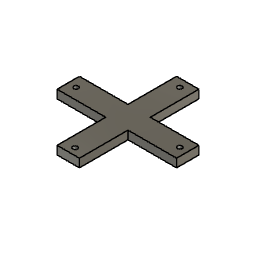
Base gripper v1 (Autodesk Fusion 360 design; units mm, degrees)
Autodesk Fusion 360 part; units mm, degrees
note: some values were not read from the file. Set by a fixed rule: which face or edge a step refers to.
sketch "Esboço1" plane through (0, 0, 0) normal (0, 0, 1) x (1, 0, 0)
  line L0 (12, 64.25) -> (-12, 64.25)
  line L1 (-12, 64.25) -> (-12, -64.25)
  line L2 (-12, -64.25) -> (12, -64.25)
  line L3 (12, -64.25) -> (12, 64.25)
  line L4 (12, 64.25) -> (-12, -64.25) construction
  line L5 (-12, 64.25) -> (12, -64.25) construction
  line L6 (64.25, 12) -> (-64.25, 12)
  line L7 (-64.25, 12) -> (-64.25, -12)
  line L8 (-64.25, -12) -> (64.25, -12)
  line L9 (64.25, -12) -> (64.25, 12)
  line L10 (64.25, 12) -> (-64.25, -12) construction
  line L11 (-64.25, 12) -> (64.25, -12) construction
  circle A0 centre (0, 0) radius 1.5
  line L12 (40, 1) -> (-40, 1)
  line L13 (-40, 1) -> (-40, -1)
  line L14 (-40, -1) -> (40, -1)
  line L15 (40, -1) -> (40, 1)
  line L16 (40, 1) -> (-40, -1) construction
  line L17 (-40, 1) -> (40, -1) construction
  line L18 (1, 40) -> (-1, 40)
  line L19 (-1, 40) -> (-1, -40)
  line L20 (-1, -40) -> (1, -40)
  line L21 (1, -40) -> (1, 40)
  line L22 (1, 40) -> (-1, -40) construction
  line L23 (-1, 40) -> (1, -40) construction
  line L24 (46.5, 6.5) -> (-46.5, 6.5)
  line L25 (-46.5, 6.5) -> (-46.5, -6.5)
  line L26 (-46.5, -6.5) -> (46.5, -6.5)
  line L27 (46.5, -6.5) -> (46.5, 6.5)
  line L28 (46.5, 6.5) -> (-46.5, -6.5) construction
  line L29 (-46.5, 6.5) -> (46.5, -6.5) construction
  line L30 (6.5, 46.5) -> (-6.5, 46.5)
  line L31 (-6.5, 46.5) -> (-6.5, -46.5)
  line L32 (-6.5, -46.5) -> (6.5, -46.5)
  line L33 (6.5, -46.5) -> (6.5, 46.5)
  line L34 (6.5, 46.5) -> (-6.5, -46.5) construction
  line L35 (-6.5, 46.5) -> (6.5, -46.5) construction
  line L36 (-64.25, 12) -> (64.25, 12)
  line L37 (64.25, 12) -> (64.25, 10)
  line L38 (64.25, 10) -> (-64.25, 10)
  line L39 (-64.25, 10) -> (-64.25, 12)
  line L40 (-64.25, -12) -> (64.25, -12)
  line L41 (64.25, -12) -> (64.25, -10)
  line L42 (64.25, -10) -> (-64.25, -10)
  line L43 (-64.25, -10) -> (-64.25, -12)
  line L44 (-64.25, 12) -> (-62.25, 12)
  line L45 (-62.25, 12) -> (-62.25, -12)
  line L46 (-62.25, -12) -> (-64.25, -12)
  line L47 (-64.25, -12) -> (-64.25, 12)
  line L48 (64.25, 12) -> (62.25, 12)
  line L49 (62.25, 12) -> (62.25, -12)
  line L50 (62.25, -12) -> (64.25, -12)
  line L51 (64.25, -12) -> (64.25, 12)
  line L52 (-12, 64.25) -> (-10, 64.25)
  line L53 (-10, 64.25) -> (-10, 10)
  line L54 (-10, 10) -> (-12, 10)
  line L55 (-12, 10) -> (-12, 64.25)
  line L56 (12, 64.25) -> (-12, 64.25)
  line L57 (-12, 64.25) -> (-12, 62.25)
  line L58 (-12, 62.25) -> (12, 62.25)
  line L59 (12, 62.25) -> (12, 64.25)
  line L60 (12, 64.25) -> (10, 64.25)
  line L61 (10, 64.25) -> (10, 12)
  line L62 (10, 12) -> (12, 12)
  line L63 (12, 12) -> (12, 64.25)
  line L64 (-12, -64.25) -> (-10, -64.25)
  line L65 (-10, -64.25) -> (-10, -10)
  line L66 (-10, -10) -> (-12, -10)
  line L67 (-12, -10) -> (-12, -64.25)
  line L68 (12, -64.25) -> (10, -64.25)
  line L69 (10, -64.25) -> (10, -10)
  line L70 (10, -10) -> (12, -10)
  line L71 (12, -10) -> (12, -64.25)
  line L72 (-12, -64.25) -> (12, -64.25)
  line L73 (12, -64.25) -> (12, -62.25)
  line L74 (12, -62.25) -> (-12, -62.25)
  line L75 (-12, -62.25) -> (-12, -64.25)
  line L76 (10, 12) -> (10, 10)
  dimension "d1" = 24
  dimension "d2" = 128.5
  dimension "d3" = 128.5
  dimension "d4" = 24
  dimension "d5" = 3
  dimension "d6" = 80
  dimension "d7" = 2
  dimension "d8" = 80
  dimension "d11" = 93
  dimension "d12" = 13
  dimension "d13" = 13
  dimension "d14" = 93
  dimension "d15" = 2
  dimension "d16" = 2
  dimension "d17" = 2
  dimension "d18" = 2
  dimension "d19" = 2
  dimension "d20" = 2
  dimension "d21" = 2
  dimension "d22" = 2
  dimension "d23" = 2
  constraint horizontal L0
  constraint perpendicular L0 L1
  constraint parallel L0 L2
  constraint parallel L1 L3
  constraint coincident L4 A0.centre
  constraint coincident L5 A0.centre
  constraint coincident A0.centre origin
  constraint horizontal L6
  constraint perpendicular L6 L7
  constraint parallel L6 L8
  constraint parallel L7 L9
  constraint coincident L10 A0.centre
  constraint coincident L11 A0.centre
  constraint horizontal L12
  constraint perpendicular L12 L13
  constraint parallel L12 L14
  constraint parallel L13 L15
  constraint coincident L16 A0.centre
  constraint coincident L17 A0.centre
  constraint horizontal L18
  constraint perpendicular L18 L19
  constraint parallel L18 L20
  constraint parallel L19 L21
  constraint coincident L22 A0.centre
  constraint coincident L23 A0.centre
  constraint horizontal L24
  constraint perpendicular L24 L25
  constraint parallel L24 L26
  constraint parallel L25 L27
  constraint coincident L28 A0.centre
  constraint coincident L29 A0.centre
  constraint horizontal L30
  constraint perpendicular L30 L31
  constraint parallel L30 L32
  constraint parallel L31 L33
  constraint coincident L34 A0.centre
  constraint coincident L35 A0.centre
  constraint horizontal L36
  constraint vertical L37
  constraint horizontal L38
  constraint vertical L39
  constraint horizontal L40
  constraint vertical L41
  constraint horizontal L42
  constraint vertical L43
  constraint horizontal L44
  constraint vertical L45
  constraint horizontal L46
  constraint vertical L47
  constraint horizontal L48
  constraint vertical L49
  constraint horizontal L50
  constraint vertical L51
  constraint horizontal L52
  constraint vertical L53
  constraint horizontal L54
  constraint vertical L55
  constraint coincident L38 L53.end
  constraint horizontal L56
  constraint vertical L57
  constraint horizontal L58
  constraint vertical L59
  constraint horizontal L60
  constraint vertical L61
  constraint horizontal L62
  constraint vertical L63
  constraint horizontal L64
  constraint vertical L65
  constraint horizontal L66
  constraint vertical L67
  constraint horizontal L68
  constraint vertical L69
  constraint horizontal L70
  constraint vertical L71
  constraint horizontal L72
  constraint vertical L73
  constraint horizontal L74
  constraint vertical L75
  constraint coincident L38 L76.end
  constraint perpendicular L38 L76
  measures "d1" distance of L0.start L0.end
  measures "d2" distance of L0.start L2.end
  measures "d3" distance of L7.end L8.end
  measures "d4" distance of L6.start L8.end
  measures "d5" diameter of A0
  measures "d6" distance of L13.end L14.end
  measures "d7" distance of L12.start L14.end
  measures "d8" distance of L18.end L19.end
  measures "d11" distance of L25.end L26.end
  measures "d12" distance of L24.end L25.end
  measures "d13" distance of L30.start L30.end
  measures "d14" distance of L30.start L32.end
  measures "d15" distance of L6.end L38.end
  measures "d16" distance of L7.end L42.end
  measures "d17" distance of L6.end L44.end
  measures "d18" distance of L6.start L48.end
  measures "d19" distance of L0.start L58.end
  measures "d20" distance of L0.start L60.end
  measures "d21" distance of L1.end L64.end
  measures "d22" distance of L2.end L68.end
  measures "d23" distance of L1.end L74.end
extrude "Extrusão1" add sketch "Esboço1" along normal blind 2 makes body 1
extrude "Extrusão2" add sketch "Esboço1" against normal blind 3 contours L6 L30 L31 L33 L36 L53 L58 L61 | L6 L33 L36 L38 L76 | L3 L24 L26 L27 L38 L42 L49 | L3 L24 L33 L38 | L6 L31 L36 L38 L53 | L1 L24 L31 L38 L54 | L1 L24 L25 L26 L38 L42 L45 | L3 L26 L33 L42 L70 | L8 L33 L40 L42 L69 | L8 L31 L32 L33 L40 L65 L69 L74 | L1 L26 L31 L42 L66 | L8 L31 L40 L42 L65 bodies 1
extrude "Extrusão3" add sketch "Esboço1" against normal blind 6 contours L0 L3 L56 L58 L59 L60 L61 L63 | L0 L53 L56 L58 L61 | L3 L6 L36 L58 L61 L62 L63 | L0 L1 L52 L53 L55 L56 L57 L58 | L3 L6 L36 L38 L49 | L3 L6 L36 L38 L62 L76 | L1 L6 L36 L53 L55 L58 | L6 L9 L36 L37 L38 L48 L49 L51 | L1 L6 L36 L38 L53 L54 L55 | L9 L38 L42 L49 L51 | L1 L6 L36 L38 L45 L55 | L3 L8 L40 L42 L49 L71 | L8 L9 L40 L41 L42 L49 L50 L51 | L6 L7 L36 L38 L39 L44 L45 L47 | L3 L8 L40 L42 L69 L70 L71 | L7 L38 L42 L45 L47 | L3 L8 L40 L69 L71 L74 | L7 L8 L40 L42 L43 L45 L46 L47 | L1 L8 L40 L42 L45 L67 | L2 L3 L68 L69 L71 L72 L73 L74 | L1 L8 L40 L42 L65 L66 L67 | L2 L65 L69 L72 L74 | L1 L8 L40 L65 L67 L74 | L1 L2 L64 L65 L67 L72 L74 L75 bodies 1
sketch "Esboço2" plane through (0, 0, 0) normal (0, 0, -1) x (1, 0, 0)
  line L0 (6.5, 46.5) -> (-6.5, 46.5)
  line L1 (-6.5, 46.5) -> (-6.5, 6.5)
  line L2 (-6.5, 6.5) -> (-46.5, 6.5)
  line L3 (-46.5, 6.5) -> (-46.5, -6.5)
  line L4 (-46.5, -6.5) -> (-6.5, -6.5)
  line L5 (-6.5, -6.5) -> (-6.5, -46.5)
  line L6 (-6.5, -46.5) -> (6.5, -46.5)
  line L7 (6.5, -46.5) -> (6.5, -6.5)
  line L8 (6.5, -6.5) -> (46.5, -6.5)
  line L9 (46.5, -6.5) -> (46.5, 6.5)
  line L10 (46.5, 6.5) -> (6.5, 6.5)
  line L11 (6.5, 6.5) -> (6.5, 46.5)
  line L12 (3, 45) -> (-3, 45)
  line L13 (-3, 45) -> (-3, -45)
  line L14 (-3, -45) -> (3, -45)
  line L15 (3, -45) -> (3, 45)
  line L16 (3, 45) -> (-3, -45) construction
  line L17 (-3, 45) -> (3, -45) construction
  line L18 (45, 3) -> (-45, 3)
  line L19 (-45, 3) -> (-45, -3)
  line L20 (-45, -3) -> (45, -3)
  line L21 (45, -3) -> (45, 3)
  line L22 (45, 3) -> (-45, -3) construction
  line L23 (-45, 3) -> (45, -3) construction
  line L24 (-3, 3) -> (-3, 10) construction
  line L25 (0, 0) -> (0, 75) construction
  line L26 (0, 0) -> (0, -75) construction
  line L27 (0, 0) -> (-80, 0) construction
  line L28 (0, 0) -> (91.9976, 0) construction
  line L29 (-3, 10) -> (0, 10) construction
  line L30 (5, -67.1453) -> (-5, -67.1453) construction
  line L31 (-5, -67.1453) -> (-5, 67.1453) construction
  line L32 (-5, 67.1453) -> (5, 67.1453) construction
  line L33 (5, 67.1453) -> (5, -67.1453)
  line L34 (5, -67.1453) -> (-5, 67.1453) construction
  line L35 (-5, -67.1453) -> (5, 67.1453) construction
  line L36 (80.4505, 5) -> (-80.4505, 5) construction
  line L37 (-80.4505, 5) -> (-80.4505, -5) construction
  line L38 (-80.4505, -5) -> (80.4505, -5) construction
  line L39 (80.4505, -5) -> (80.4505, 5) construction
  line L40 (80.4505, 5) -> (-80.4505, -5) construction
  line L41 (-80.4505, 5) -> (80.4505, -5) construction
  line L42 (-5, 3) -> (-5, 10) construction
  line L43 (-5, 10) -> (5, 10)
  line L44 (5, 10) -> (5, 15)
  line L45 (5, 15) -> (-5, 15)
  line L46 (-5, 15) -> (-5, 10)
  line L47 (-5, 15) -> (5, 10) construction
  line L48 (5, 13.5) -> (-5, 13.5)
  line L49 (-5, 13.5) -> (-5, 11.5)
  line L50 (-5, 11.5) -> (5, 11.5)
  line L51 (5, 11.5) -> (5, 13.5)
  line L52 (5, 13.5) -> (-5, 11.5) construction
  line L53 (-5, 13.5) -> (5, 11.5) construction
  line L54 (-5, 15) -> (-5, 18.2)
  line L55 (-5, 18.2) -> (5, 18.2)
  line L56 (5, 18.2) -> (5, 23.7)
  line L57 (5, 23.7) -> (-5, 23.7)
  line L58 (-5, 23.7) -> (-5, 18.2)
  line L59 (5, 22.25) -> (-5, 22.25)
  line L60 (-5, 22.25) -> (-5, 19.75)
  line L61 (-5, 19.75) -> (5, 19.75)
  line L62 (5, 19.75) -> (5, 22.25)
  line L63 (5, 22.25) -> (-5, 19.75) construction
  line L64 (-5, 22.25) -> (5, 19.75) construction
  line L65 (-5, 23.7) -> (-5, 27.5)
  line L66 (-5, 27.5) -> (5, 27.5)
  line L67 (5, 27.5) -> (5, 32.5)
  line L68 (5, 32.5) -> (-5, 32.5)
  line L69 (-5, 32.5) -> (-5, 27.5)
  line L70 (5, 31.25) -> (-5, 31.25)
  line L71 (-5, 31.25) -> (-5, 28.75)
  line L72 (-5, 28.75) -> (5, 28.75)
  line L73 (5, 28.75) -> (5, 31.25)
  line L74 (5, 31.25) -> (-5, 28.75) construction
  line L75 (-5, 31.25) -> (5, 28.75) construction
  line L76 (-5, 32.5) -> (-5, 36.5)
  line L77 (-5, 36.5) -> (5, 36.5)
  line L78 (5, 36.5) -> (5, 44)
  line L79 (5, 44) -> (-5, 44)
  line L80 (-5, 44) -> (-5, 36.5)
  line L81 (-5, 44) -> (5, 36.5) construction
  line L82 (5, 43.25) -> (-5, 43.25)
  line L83 (-5, 43.25) -> (-5, 37.25)
  line L84 (-5, 37.25) -> (5, 37.25)
  line L85 (5, 37.25) -> (5, 43.25)
  line L86 (5, 43.25) -> (-5, 37.25) construction
  line L87 (-5, 43.25) -> (5, 37.25) construction
  line L88 (45, 1.5) -> (-45, 1.5)
  line L89 (-45, 1.5) -> (-45, -1.5)
  line L90 (-45, -1.5) -> (45, -1.5)
  line L91 (45, -1.5) -> (45, 1.5)
  line L92 (45, 1.5) -> (-45, -1.5) construction
  line L93 (-45, 1.5) -> (45, -1.5) construction
  line L94 (1.5, 45) -> (-1.5, 45)
  line L95 (-1.5, 45) -> (-1.5, -45)
  line L96 (-1.5, -45) -> (1.5, -45)
  line L97 (1.5, -45) -> (1.5, 45)
  line L98 (1.5, 45) -> (-1.5, -45) construction
  line L99 (-1.5, 45) -> (1.5, -45) construction
  point P0 (0, 12.5)
  point P1 (0, 21)
  point P2 (0, 30)
  point P3 (0, 40.25)
  dimension "d28" = 6
  dimension "d29" = 90
  dimension "d30" = 90
  dimension "d31" = 7
  dimension "d33" = 6
  dimension "d34" = 10
  dimension "d35" = 10
  dimension "d36" = 5
  dimension "d37" = 2
  dimension "d38" = 3.2
  dimension "d39" = 5.5
  dimension "d40" = 2.5
  dimension "d41" = 3.8
  dimension "d42" = 5
  dimension "d43" = 2.5
  dimension "d44" = 4
  dimension "d45" = 7.5
  dimension "d46" = 6
  dimension "d47" = 3
  dimension "d48" = 3
  constraint horizontal L12
  constraint perpendicular L12 L13
  constraint parallel L12 L14
  constraint parallel L13 L15
  constraint coincident L16 L25.start
  constraint coincident L17 L25.start
  constraint coincident L25.start L26.start
  constraint horizontal L18
  constraint perpendicular L18 L19
  constraint parallel L18 L20
  constraint parallel L19 L21
  constraint coincident L22 L25.start
  constraint coincident L23 L25.start
  constraint coincident L13 L24.start
  constraint coincident L18 L24.start
  constraint perpendicular L18 L24
  constraint perpendicular L12 L25
  constraint parallel L15 L26
  constraint perpendicular L3 L27
  constraint perpendicular L9 L28
  constraint coincident L25 L29.end
  constraint perpendicular L25 L29
  constraint horizontal L30
  constraint perpendicular L30 L31
  constraint parallel L30 L32
  constraint parallel L31 L33
  constraint coincident L34 L25.start
  constraint coincident L35 L25.start
  constraint horizontal L36
  constraint perpendicular L36 L37
  constraint parallel L36 L38
  constraint parallel L37 L39
  constraint coincident L40 L25.start
  constraint coincident L41 L25.start
  constraint coincident L18 L42.start
  constraint coincident L31 L42.start
  constraint coincident L31 L42.end
  constraint horizontal L43
  constraint vertical L44
  constraint horizontal L45
  constraint vertical L46
  constraint horizontal L48
  constraint perpendicular L48 L49
  constraint parallel L48 L50
  constraint parallel L49 L51
  constraint coincident L52 P0
  constraint coincident L53 P0
  constraint midpoint L47 P0
  constraint perpendicular L45 L54
  constraint horizontal L55
  constraint vertical L56
  constraint horizontal L57
  constraint vertical L58
  constraint horizontal L59
  constraint perpendicular L59 L60
  constraint parallel L59 L61
  constraint parallel L60 L62
  constraint coincident L63 P1
  constraint coincident L64 P1
  constraint coincident L25 P1
  constraint perpendicular L57 L65
  constraint horizontal L66
  constraint vertical L67
  constraint horizontal L68
  constraint vertical L69
  constraint horizontal L70
  constraint perpendicular L70 L71
  constraint parallel L70 L72
  constraint parallel L71 L73
  constraint coincident L74 P2
  constraint coincident L75 P2
  constraint coincident L67 L70.start
  constraint coincident L33 L70.start
  constraint coincident L25 P2
  constraint perpendicular L68 L76
  constraint horizontal L77
  constraint vertical L78
  constraint horizontal L79
  constraint vertical L80
  constraint horizontal L82
  constraint perpendicular L82 L83
  constraint parallel L82 L84
  constraint parallel L83 L85
  constraint coincident L86 P3
  constraint coincident L87 P3
  constraint coincident L78 L82.start
  constraint coincident L33 L82.start
  constraint midpoint L81 P3
  constraint horizontal L88
  constraint perpendicular L88 L89
  constraint parallel L88 L90
  constraint parallel L89 L91
  constraint coincident L92 L25.start
  constraint coincident L93 L25.start
  constraint coincident L21 L88.start
  constraint horizontal L94
  constraint perpendicular L94 L95
  constraint parallel L94 L96
  constraint parallel L95 L97
  constraint coincident L98 L25.start
  constraint coincident L99 L25.start
  measures "d28" distance of L13.end L14.end
  measures "d29" distance of L12.start L14.end
  measures "d30" distance of L19.end L20.end
  measures "d31" distance of L24.start L24.end
  measures "d33" distance of L18.end L19.end
  measures "d34" distance of L31.end L32.end
  measures "d35" distance of L36.end L37.end
  measures "d36" distance of L42.end L45.end
  measures "d37" distance of L48.end L49.end
  measures "d38" distance of L45.end L54.end
  measures "d39" distance of L54.end L57.end
  measures "d40" distance of L59.end L60.end
  measures "d41" distance of L57.end L65.end
  measures "d42" distance of L65.end L68.end
  measures "d43" distance of L70.end L71.end
  measures "d44" distance of L68.end L76.end
  measures "d45" distance of L76.end L79.end
  measures "d46" distance of L82.end L83.end
  measures "d47" distance of L88.end L89.end
  measures "d48" distance of L95.end L96.end
extrude "Extrusão4" add sketch "Esboço2" along normal blind 3 separate body contours L15 L33 L78 L79 L82 | L15 L33 L78 L82 L84 L85 | L15 L79 L82 L97 | L15 L33 L77 L78 L84 | L15 L82 L84 L97 | L79 L82 L95 L97 | L15 L77 L84 L97 | L82 L84 L95 L97 | L13 L79 L82 L95 | L15 L33 L67 L68 L70 | L15 L68 L77 L97 | L77 L84 L95 L97 | L13 L82 L84 L95 | L13 L79 L80 L82 | L15 L33 L67 L70 L72 L73 | L15 L68 L70 L97 | L68 L77 L95 L97 | L13 L77 L84 L95 | L13 L80 L82 L83 L84 | L15 L33 L66 L67 L72 | L15 L70 L72 L97 | L68 L70 L95 L97 | L13 L68 L77 L95 | L13 L77 L80 L84 | L15 L66 L72 L97 | L70 L72 L95 L97 | L13 L68 L70 L95 | L15 L33 L56 L57 L59 | L15 L57 L66 L97 | L66 L72 L95 L97 | L13 L70 L72 L95 | L13 L68 L69 L70 | L15 L33 L56 L59 L61 L62 | L15 L57 L59 L97 | L57 L66 L95 L97 | L13 L66 L72 L95 | L13 L69 L70 L71 L72 | L15 L18 L43 L97 | L15 L33 L43 L44 L50 | L15 L33 L55 L56 L61 | L15 L59 L61 L97 | L57 L59 L95 L97 | L13 L57 L66 L95 | L13 L66 L69 L72 | L15 L43 L50 L97 | L18 L43 L95 L97 | L15 L33 L44 L48 L50 L51 | L15 L55 L61 L97 | L59 L61 L95 L97 | L13 L57 L59 L95 | L15 L48 L50 L97 | L43 L50 L95 L97 | L13 L18 L43 L95 | L15 L33 L44 L45 L48 | L15 L45 L55 L97 | L55 L61 L95 L97 | L13 L59 L61 L95 | L13 L57 L58 L59 | L15 L45 L48 L97 | L48 L50 L95 L97 | L13 L43 L50 L95 | L45 L55 L95 L97 | L13 L55 L61 L95 | L13 L58 L59 L60 L61 | L45 L48 L95 L97 | L13 L48 L50 L95 | L13 L43 L46 L50 | L13 L45 L55 L95 | L13 L55 L58 L61 | L13 L45 L48 L95 | L13 L46 L48 L49 L50 | L13 L45 L46 L48 makes body 2
mirror "Espelhar1" about plane through (0, 0, 0) normal (0, 0, 1) of bodies 2 merged
extrude "Extrusão5" add sketch "Esboço2" along normal blind 5 separate body contours L79 L82 L95 L97 | L82 L84 L95 L97 | L77 L84 L95 L97 | L68 L77 L95 L97 | L68 L70 L95 L97 | L70 L72 L95 L97 | L14 L20 L95 L96 L97 | L20 L90 L95 L97 | L66 L72 L95 L97 | L88 L90 L95 L97 | L57 L66 L95 L97 | L18 L88 L95 L97 | L57 L59 L95 L97 | L18 L43 L95 L97 | L59 L61 L95 L97 | L43 L50 L95 L97 | L55 L61 L95 L97 | L48 L50 L95 L97 | L45 L55 L95 L97 | L45 L48 L95 L97 makes body 3
extrude "Extrusão6" add sketch "Esboço2" along normal blind 10 separate body contours L15 L33 L78 L82 L84 L85 | L15 L82 L84 L97 | L82 L84 L95 L97 | L13 L82 L84 L95 | L15 L33 L67 L70 L72 L73 | L13 L80 L82 L83 L84 | L15 L70 L72 L97 | L70 L72 L95 L97 | L13 L70 L72 L95 | L15 L33 L56 L59 L61 L62 | L13 L69 L70 L71 L72 | L15 L59 L61 L97 | L15 L33 L44 L48 L50 L51 | L59 L61 L95 L97 | L15 L48 L50 L97 | L13 L59 L61 L95 | L48 L50 L95 L97 | L13 L58 L59 L60 L61 | L13 L48 L50 L95 | L13 L46 L48 L49 L50 makes body 4 at (-1.6667, -19.75, -3.3333) makes body 5 at (-1.6667, -28.75, -3.3333) makes body 6 at (-1.6667, -11.5, -3.3333) makes body 7 at (-1.6667, -37.25, -3.3333)
combine "Combinar1" operation add target body 7 tool bodies 6 3 4 5 2
copy_body "Copiar e colar corpos1" bodies 7 makes body 8
move_body "Mover1" bodies 8 to x (0, 1, 0) y (-1, 0, 0) z (0, 0, 1) at (1, 0, 0)
extrude "Extrusão7" add 1 faces at (-0.5, -43.25, -8.3333) along direction (0, -1, 0) blind 0.75 on bodies 7 bodies 7
extrude "Extrusão8" add 1 faces at (44.25, -0.5, -8.3333) along direction (1, 0, 0) blind 0.75 on bodies 8 bodies 8
copy_body "Copiar e colar corpos2" bodies 8 makes body 9
move_body "Mover2" bodies 9 to x (0, 1, 0) y (-1, 0, 0) z (0, 0, 1) at (0, 0, 0)
copy_body "Copiar e colar corpos3" bodies 8 makes body 10
move_body "Mover3" bodies 10 to x (-1, 0, 0) y (0, -1, 0) z (0, 0, 1) at (0, 0, 0)
extrude "Extrusão9" add 1 faces at (4, 0.5, 2) along direction (-1, 0, 0) blind 8.5 on bodies 8 bodies 8 1 7 9 10
extrude "Extrusão10" add 1 faces at (1.6667, -57.5, 2) along direction (0, 0, 1) blind 1 on bodies 8 bodies 8
extrude "Extrusão11" add 2 faces at (2, 4, -1) (-2, 4, -2) along direction (0, -1, 0) blind 1 on bodies 8 bodies 8
sketch "Esboço3" plane through (0, 0, -5) normal (0, 0, -1) x (1, 0, 0)
  line L0 (1.5, 1.5) -> (1.5, 11.5)
  line L1 (1.5, 11.5) -> (-1.5, 11.5)
  line L2 (-1.5, 11.5) -> (-1.5, 1.5)
  line L3 (-1.5, 1.5) -> (-12.5, 1.5)
  line L4 (-12.5, 1.5) -> (-12.5, -1.5)
  line L5 (-12.5, -1.5) -> (-1.5, -1.5)
  line L6 (-1.5, -1.5) -> (-1.5, -12.5)
  line L7 (-1.5, -12.5) -> (1.5, -12.5)
  line L8 (1.5, -12.5) -> (1.5, -1.5)
  line L9 (1.5, -1.5) -> (12.5, -1.5)
  line L10 (12.5, -1.5) -> (12.5, 1.5)
  line L11 (12.5, 1.5) -> (1.5, 1.5)
  circle A0 centre (0, 0) radius 1.5
  dimension "d67" = 3
  constraint coincident A0.centre origin
  measures "d67" diameter of A0
extrude "Extrusão12" add sketch "Esboço3" along normal blind 10 contours A0 bodies 8
fillet "Arredondamento1" radius 0.5 1 edges at (-1.3985, -0.5424, -5) on bodies 8
extrude "Extrusão13" add 1 faces at (0.567, 0.5383, -15) along direction (0, 0, -1) blind 2 on bodies 8 bodies 8
sketch "Esboço4" plane through (0, 0, -3) normal (0, 0, -1) x (1, 0, 0)
  line L0 (6.5, 46.5) -> (6.5, 6.5)
  line L1 (6.5, 6.5) -> (46.5, 6.5)
  line L2 (46.5, 6.5) -> (46.5, -6.5)
  line L3 (46.5, -6.5) -> (6.5, -6.5)
  line L4 (6.5, -6.5) -> (6.5, -46.5)
  line L5 (6.5, -46.5) -> (-6.5, -46.5)
  line L6 (-6.5, -46.5) -> (-6.5, -6.5)
  line L7 (-6.5, -6.5) -> (-46.5, -6.5)
  line L8 (-46.5, -6.5) -> (-46.5, 6.5)
  line L9 (-46.5, 6.5) -> (-6.5, 6.5)
  line L10 (-6.5, 6.5) -> (-6.5, 46.5)
  line L11 (-6.5, 46.5) -> (6.5, 46.5)
  line L12 (-10, -10) -> (-10, -62.25)
  line L13 (-10, -62.25) -> (10, -62.25)
  line L14 (10, -62.25) -> (10, -10)
  line L15 (10, -10) -> (62.25, -10)
  line L16 (62.25, -10) -> (62.25, 10)
  line L17 (62.25, 10) -> (10, 10)
  line L18 (10, 10) -> (10, 62.25)
  line L19 (10, 62.25) -> (-10, 62.25)
  line L20 (-10, 62.25) -> (-10, 10)
  line L21 (-10, 10) -> (-62.25, 10)
  line L22 (-62.25, 10) -> (-62.25, -10)
  line L23 (-62.25, -10) -> (-10, -10)
  line L24 (-62.25, 0) -> (-61.75, 0)
  line L25 (62.25, 0) -> (61.75, 0)
  line L26 (-61.75, 0) -> (-61.75, 10) construction
  line L27 (-61.75, 0) -> (-61.75, -10) construction
  line L28 (-61.75, -10) -> (-49.75, -10) construction
  line L29 (-49.75, -10) -> (-49.75, 10) construction
  line L30 (-49.75, 10) -> (-61.75, 10) construction
  line L31 (-61.75, 10) -> (-61.75, -10)
  line L32 (-61.75, 10) -> (-49.75, -10) construction
  circle A0 centre (-55.75, 0) radius 2.5
  line L33 (0, 62.25) -> (0, 61.75)
  line L34 (0, 61.75) -> (-10, 61.75)
  line L35 (-10, 61.75) -> (10, 61.75)
  line L36 (10, 61.75) -> (10, 51.9531)
  line L37 (10, 51.9531) -> (-10, 51.9531) construction
  line L38 (-10, 51.9531) -> (-10, 61.75)
  line L39 (-10, 61.75) -> (10, 51.9531) construction
  circle A1 centre (0, 56.8516) radius 2.5
  line L40 (61.75, 0) -> (61.75, -10)
  line L41 (61.75, -10) -> (49.75, -10)
  line L42 (49.75, -10) -> (49.75, 10)
  line L43 (49.75, 10) -> (61.75, 10)
  line L44 (61.75, 10) -> (61.75, -10)
  line L45 (49.75, 10) -> (61.75, -10) construction
  circle A2 centre (55.75, 0) radius 2.5
  line L46 (0, -62.25) -> (0, -61.75)
  line L47 (0, -61.75) -> (-10, -61.75)
  line L48 (-10, -61.75) -> (10, -61.75) construction
  line L49 (10, -61.75) -> (10, -49.75) construction
  line L50 (10, -49.75) -> (-10, -49.75) construction
  line L51 (-10, -49.75) -> (-10, -61.75) construction
  line L52 (-10, -49.75) -> (10, -61.75) construction
  circle A3 centre (0, -55.75) radius 2.5
  dimension "d74" = 0.5
  dimension "d75" = 0.5
  dimension "d76" = 12
  dimension "d77" = 5
  dimension "d78" = 0.5
  dimension "d79" = 5
  dimension "d80" = 12
  dimension "d81" = 5
  dimension "d82" = 0.5
  dimension "d83" = 12
  dimension "d84" = 5
  constraint midpoint L22 L24.start
  constraint horizontal L24
  constraint midpoint L16 L25.start
  constraint horizontal L25
  constraint perpendicular L24 L26
  constraint coincident L23 L27.end
  constraint perpendicular L23 L27
  constraint horizontal L28
  constraint vertical L29
  constraint horizontal L30
  constraint vertical L31
  constraint midpoint L32 A0.centre
  constraint midpoint L19 L33.start
  constraint vertical L33
  constraint coincident L20 L34.end
  constraint perpendicular L20 L34
  constraint horizontal L35
  constraint vertical L36
  constraint horizontal L37
  constraint vertical L38
  constraint coincident L18 L36.end
  constraint midpoint L39 A1.centre
  constraint coincident L15 L40.end
  constraint perpendicular L15 L40
  constraint horizontal L41
  constraint vertical L42
  constraint horizontal L43
  constraint vertical L44
  constraint midpoint L45 A2.centre
  constraint midpoint L13 L46.start
  constraint vertical L46
  constraint coincident L12 L47.end
  constraint perpendicular L12 L47
  constraint horizontal L48
  constraint vertical L49
  constraint horizontal L50
  constraint vertical L51
  constraint midpoint L52 A3.centre
  measures "d74" distance of L24.start L24.end
  measures "d75" distance of L25.start L25.end
  measures "d76" distance of L27.end L28.end
  measures "d77" diameter of A0
  measures "d78" distance of L33.start L33.end
  measures "d79" diameter of A1
  measures "d80" distance of L40.end L41.end
  measures "d81" diameter of A2
  measures "d82" distance of L46.start L46.end
  measures "d83" distance of L47.end L50.end
  measures "d84" diameter of A3
extrude "Extrusão14" cut sketch "Esboço4" against normal blind 9 contours A0 | A1 | A2 | A3 bodies 8
